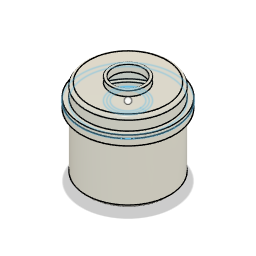
V2-CPAP-normal_cover_v3 (Autodesk Fusion 360 archive; units mm, degrees)
design "cpap motor"
Autodesk Fusion 360 part; units mm, degrees
sketch "Sketch1" plane through (0, 0, 0) normal (0, 1, 0) x (1, 0, 0)
  circle A0 centre (-0.1554, 0) radius 26.5
  circle A1 centre (-0.1554, 0) radius 29.5
  circle A2 centre (-0.1554, 0) radius 11
  circle A3 centre (-0.1554, 0) radius 8
  circle A4 centre (-0.1554, 0) radius 9.5
  dimension "d1" = 53
  dimension "d2" = 59
  dimension "d3" = 22
  dimension "d4" = 16
  dimension "d11" = 19
  constraint concentric A0 A1
  constraint concentric A1 A2
  constraint concentric A1 A3
  constraint concentric A3 A4
  measures "d1" diameter of A0
  measures "d2" diameter of A1
  measures "d3" diameter of A2
  measures "d4" diameter of A3
  measures "d11" diameter of A4
extrude "Extrude1" add sketch "Sketch1" along normal blind 14 contours A2 | A4 makes body 1
extrude "Extrude2" add sketch "Sketch1" along normal blind 2 contours A0 | A1 bodies 1
extrude "Extrude3" add sketch "Sketch1" along normal blind 10 contours A0 bodies 1
extrude "Extrude4" cut sketch "Sketch1" along normal blind 14 contours A4 bodies 1
extrude "Extrude5" add sketch "Sketch1" against normal blind 4 separate body contours A0 | A1 makes body 2
extrude "Extrude6" add sketch "Sketch1" against normal blind 40 contours A0 | A2 | A4 bodies 2
extrude "Extrude7" add 1 faces at (20.0793, -40, 1.3165) along direction (0, -1, 0) blind 4 on bodies 2 bodies 2
ref_plane "WorkPlane1" through (0, 0, 0) normal (0, 0, 1) x (1, 0, 0)
sketch "Sketch2" plane through (0, 0, 0) normal (0, 0, 1) x (1, 0, 0)
  line L0 (30.4771, -40.0518) -> (30.4771, -50)
  line L1 (30.4771, -50) -> (6.4219, -50)
  arc A0 (30.4771, -40.0518) -> (6.4219, -44.7074) centre (27.6605, -89.9724) ccw
  line L2 (6.4219, -44.7074) -> (6.4219, -50)
  dimension "d21" = 100
  constraint vertical L0
  constraint perpendicular L0 L1
  constraint perpendicular L1 L2
  measures "d21" diameter of A0
revolve "Revolve1" cut sketch "Sketch2" angle 360 about axis through (-0.1554, -40, 0) along (0, 1, 0) bodies 2
fillet "Fillet1" radius 1.5 1 edges at (-24.8621, -39.9897, 9.5828) on bodies 2
fillet "Fillet2" radius 0.75 2 edges at (-9.0125, 14, -3.4353) (-10.411, 14, 3.9778) on bodies 1
fillet "Fillet3" radius 2 1 edges at (-24.8621, 10, 9.5828) on bodies 1
shell "Shell1" thickness 5 removed faces 1 at (7.8347, -29.3333, 0.3988) on bodies 2
move_face "OffsetFaces1" offset -16 1 faces at (7.8347, -3.3333, 0.3988) on bodies 2
extrude "Extrude8" cut 1 faces at (22.9219, -5, 1.1923) along direction (0, 1, 0) blind 14 on bodies 2 bodies 1
extrude "Extrude9" cut 1 faces at (17.2646, 0, -1.0681) along direction (0, 1, 0) blind 9 on bodies 1 bodies 1
ref_plane "WorkPlane2" through (-0.1554, -29.5, 0) normal (0, -1, 0) x (-1, 0, 0)
